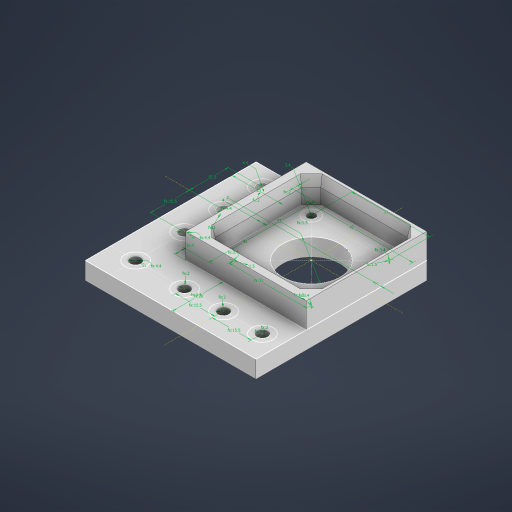
# Autodesk Inventor part: Z Stepper Holder
Saved by Autodesk Inventor 2024.2 (Build 282272000, 272)
## iProperties
Created: 2024-10-05
Part Number: Z Stepper Holder
Material: Generic
Document SubType Name: Modeling
Designer: jerem
Density: 1 g/cm^3
Appearance: Default
Author: jerem
Autodesk Inventor part; units mm, degrees
ref_plane "YZ Plane" through (0, 0, 0) normal (1, 0, 0) x (0, 1, 0)
ref_plane "XZ Plane" through (0, 0, 0) normal (0, 1, 0) x (-1, 0, 0)
ref_plane "XY Plane" through (0, 0, 0) normal (0, 0, 1) x (1, 0, 0)
sketch "Sketch1" plane through (0, 0, 0) normal (0, 1, 0) x (-1, 0, 0)
  line L0 (-21, 21) -> (21, 21)
  line L1 (21, 21) -> (21, -21)
  line L2 (21, -21) -> (-21, -21)
  line L3 (-21, -21) -> (-21, 21)
  line L4 (-21, 21) -> (21, -21) construction
  line L5 (21, 21) -> (-21, -21) construction
  circle A0 centre (15.5, -15.5) radius 1.7
  circle A1 centre (-15.5, -15.5) radius 1.7
  line L6 (15.5, -15.5) -> (-15.5, -15.5) construction
  circle A2 centre (15.5, 15.5) radius 1.7
  line L7 (15.5, 15.5) -> (-15.5, 15.5) construction
  circle A3 centre (-15.5, 15.5) radius 1.7
  line L8 (-23, 25) -> (25, 25)
  line L9 (25, 25) -> (25, -23)
  line L10 (25, -23) -> (-23, -23)
  line L11 (-23, -23) -> (-23, 25)
  circle A4 centre (0, 0) radius 11.5
  line L12 (25, 25) -> (-23, 25)
  line L13 (-23, 25) -> (-23, 45)
  line L14 (-23, 45) -> (45, 45)
  line L15 (45, 45) -> (45, -23)
  line L16 (45, -23) -> (25, -23)
  circle A5 centre (35, -15.5) radius 2.2
  circle A6 centre (35, 15.5) radius 2.2
  circle A7 centre (35, 0) radius 2.2
  circle A8 centre (-15.5, 35) radius 2.2
  circle A9 centre (0, 35) radius 2.2
  circle A10 centre (15.5, 35) radius 2.2
  line L17 (-23, 35) -> (45, 35) construction
  line L18 (35, 45) -> (35, -23) construction
  line L19 (0, -36.6) -> (0, 58.6) construction
  line L20 (58.6, 0) -> (-36.6, 0) construction
  circle A11 centre (35, 15.5) radius 4.2
  circle A12 centre (35, 0) radius 4.2
  circle A13 centre (35, -15.5) radius 4.2
  circle A14 centre (15.5, 35) radius 4.2
  circle A15 centre (0, 35) radius 4.2
  circle A16 centre (-15.5, 35) radius 4.2
  circle A17 centre (15.5, 15.5) radius 3.2
  circle A18 centre (-15.5, 15.5) radius 3.2
  circle A19 centre (-15.5, -15.5) radius 3.2
  circle A20 centre (15.5, -15.5) radius 3.2
  circle A21 centre (35, 35) radius 2.2
  circle A22 centre (35, 35) radius 4.2
  point P0 (11, 45)
  dimension "d20" = 31
  dimension "d21" = 42
  dimension "d22" = 42
  dimension "d23" = 3.4
  dimension "d24" = 3.4
  dimension "d25" = 3.4
  dimension "d26" = 31
  dimension "d27" = 3.4
  dimension "d28" = 4
  dimension "d29" = 4
  dimension "d30" = 2
  dimension "d31" = 2
  dimension "d32" = 23
  dimension "d37" = 20
  dimension "d38" = 20
  dimension "d39" = 4.4
  dimension "d40" = 4.4
  dimension "d42" = 4.4
  dimension "d43" = 4.4
  dimension "d44" = 4.4
  dimension "d45" = 4.4
  dimension "d47" = 15.5
  dimension "d48" = 15.5
  dimension "d51" = 15.5
  dimension "d52" = 15.5
  dimension "d59" = 2
  dimension "d60" = 1.5
  dimension "d61" = 1.5
  dimension "d62" = 1.5
  dimension "d63" = 1.5
  dimension "d64" = 2
  dimension "d65" = 2
  dimension "d66" = 2
  dimension "d67" = 2
  dimension "d68" = 2
  dimension "d69" = 4.4
  dimension "d70" = 2
  constraints: 38 end point, 23 centre point, 17 point on line, 7 perpendicular, 6 midpoint, 5 horizontal, 4 parallel, 2 coincident, 1 vertical
  measures "d20" distance of L6.end L6.start
  measures "d21" distance of L1.end L2.end
  measures "d22" distance of L0.end L1.end
  measures "d23" diameter of A0
  measures "d24" diameter of A1
  measures "d25" diameter of A2
  measures "d26" distance of L7.start L7.end
  measures "d27" diameter of A3
  measures "d28" distance between parallel lines of L9 L1
  measures "d29" distance between parallel lines of L8 L0
  measures "d30" distance between parallel lines of L10 L2
  measures "d31" distance between parallel lines of L11 L3
  measures "d32" diameter of A4
  measures "d37" distance between parallel lines of L9 L15
  measures "d38" distance from line of point (11, 45) L12
  measures "d39" diameter of A5
  measures "d40" diameter of A7
  measures "d42" diameter of A10
  measures "d43" diameter of A9
  measures "d44" diameter of A8
  measures "d45" diameter of A6
  measures "d47" distance of A5.centre A7.centre
  measures "d48" distance of A6.centre A7.centre
  measures "d51" distance of A9.centre A10.centre
  measures "d52" distance of A8.centre A9.centre
  measures "d59" radial gap between concentric circles of A6 A11
  measures "d60" radial gap between concentric circles of A2 A17
  measures "d61" radial gap between concentric circles of A18 A3
  measures "d62" radial gap between concentric circles of A1 A19
  measures "d63" radial gap between concentric circles of A0 A20
  measures "d64" radial gap between concentric circles of A7 A12
  measures "d65" radial gap between concentric circles of A5 A13
  measures "d66" radial gap between concentric circles of A14 A10
  measures "d67" radial gap between concentric circles of A15 A9
  measures "d68" radial gap between concentric circles of A16 A8
  measures "d69" diameter of A21
  measures "d70" radial gap between concentric circles of A21 A22
extrude "Extrusion1" add sketch "Sketch1" along normal blind 10 contours L8 L9 L10 L11
extrude "Extrusion2" add sketch "Sketch1" against normal blind 7 contours L0 L1 L2 L3 | L13 L14 L15 L16 L9 L8 | L8 L9 L10 L11 | A11 | A12 | A13 | A14 | A15 | A16 | A17 | A18 | A19 | A20 | A22
chamfer "Chamfer1" distance 3.8 angle 45 4 edges at (-21, 5, 21) (-21, 5, -21) (21, 5, -21) (21, 5, 21)
chamfer "Chamfer2" distance 1 distance2 4 8 edges at (0, 10, -21) (19.1, 10, -19.1) (21, 10, 0) (19.1, 10, 19.1) (0, 10, 21) (-21, 10, 0) (-19.1, 10, -19.1) (-19.1, 10, 19.1) measured on face at (0, 10, -21.5) measured on face at (-21.5, 10, 0) measured on face at (19.4536, 10, -19.4536) measured on face at (-19.4536, 10, -19.4536) measured on face at (21.5, 10, 0) measured on face at (19.4536, 10, 19.4536) measured on face at (-19.4536, 10, 19.4536) measured on face at (0, 10, 21.5)
extrude "Extrusion3" cut sketch "Sketch1" along normal blind 2 from surface at -7 contours A3 | A5 | A6 | A7 | A8 | A11 | A12 | A13 | A14 | A15 | A16 | A17 | A18 | A19 | A20 | A22
equation "\"d24\" = d23"
equation "\"d25\" = d23"
equation "\"d26\" = d20"
equation "\"d27\" = d23"
equation "\"d29\" = d28"
equation "\"d30\" = d31"
equation "\"d38\" = d37"
equation "\"d40\" = d39"
equation "\"d42\" = d39"
equation "\"d43\" = d39"
equation "\"d44\" = d39"
equation "\"d45\" = d39"
body "Solid1"
